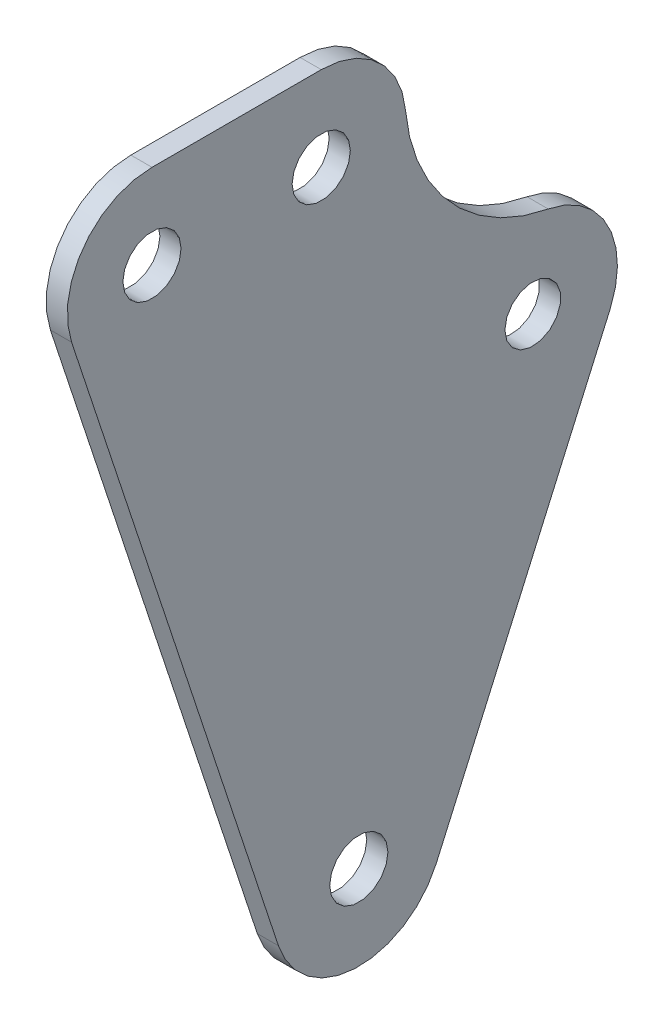
# Autodesk Inventor part: bottom_joint_gusset
Saved by Autodesk Inventor 2025 (Build 290162000, 162)
## iProperties
Created: 2024-10-13
Part Number: bottom_joint_gusset
Material: Generic
Document SubType Name: Modeling
Designer: Averey Ku
Density: 1 g/cm^3
Appearance: Default
Author: Averey Ku
Autodesk Inventor part; units mm, degrees
ref_plane "YZ Plane" through (0, 0, 0) normal (1, 0, 0) x (0, 1, 0)
ref_plane "XZ Plane" through (0, 0, 0) normal (0, 1, 0) x (-1, 0, 0)
ref_plane "XY Plane" through (0, 0, 0) normal (0, 0, 1) x (1, 0, 0)
sketch "maiin" plane through (0, 0, 0) normal (0, 0, 1) x (1, 0, 0)
  circle A0 centre (-0.0182, -20.0228) radius 2.1844
  circle A1 centre (12.6818, -20.0228) radius 2.1844
  circle A2 centre (-2.8225, 26.9672) radius 2.1844 construction
  arc A3 (-6.3396, -20.5787) -> (-0.0224, -26.3686) centre (-0.0182, -20.0228) ccw
  arc A4 (12.6776, -26.377) -> (18.7159, -18.0313) centre (12.6818, -20.0228) ccw
  arc A5 (3.2076, 28.9574) -> (-8.6291, 29.5373) centre (-2.8225, 26.9672) ccw
  arc A6 (-21.694, 0.0193) -> (-17.0461, -8.7942) centre (-15.8874, -2.5508) ccw
  circle A7 centre (-15.8874, -2.5508) radius 2.0955
  line L0 (18.7159, -18.0313) -> (3.2076, 28.9574)
  line L1 (12.6776, -26.377) -> (-0.0224, -26.3686)
  line L2 (-8.6291, 29.5373) -> (-21.694, 0.0193)
  circle A8 centre (-2.8225, 26.9672) radius 2.1844
  arc A9 (-6.3396, -20.5787) -> (-17.0461, -8.7942) centre (-19.447, -21.7313) ccw
  point P0 (3.1417, -3.9392)
  dimension "d0" = 12.7
  dimension "d1" = 12.7
  dimension "d2" = 4.191
  dimension "d3" = 4.3688
  dimension "d7" = 46.99
  measures "d0" diameter of A5
  measures "d1" diameter of A6
  measures "d2" diameter of A7
  measures "d3" diameter of A8
  measures "d7" vertical distance of A2.centre A0.centre
sketch "Sketch1" plane through (0, 0, 0) normal (1, 0, 0) x (0, 1, 0)
  circle A0 centre (0.0042, -12.7) radius 2.1844
  circle A1 centre (0, 0) radius 2.1844
  circle A2 centre (-46.9848, -15.5199) radius 2.1844 construction
  arc A3 (0.5622, -19.0212) -> (6.35, -12.7021) centre (0.0042, -12.7) ccw
  arc A4 (6.3542, -0.0021) -> (-1.9935, 6.0334) centre (0, 0) ccw
  arc A5 (-48.977, -9.4905) -> (-49.553, -21.3275) centre (-46.9848, -15.5199) ccw
  arc A6 (-20.0306, -34.3825) -> (-11.2187, -29.7316) centre (-17.4625, -28.575) ccw
  circle A7 centre (-17.4625, -28.575) radius 2.0955
  line L0 (-1.9935, 6.0334) -> (-48.977, -9.4905)
  line L1 (6.3542, -0.0021) -> (6.35, -12.7021)
  line L2 (-49.553, -21.3275) -> (-20.0306, -34.3825)
  circle A8 centre (-46.9848, -15.5199) radius 2.1844
  arc A9 (0.5622, -19.0212) -> (-11.2187, -29.7316) centre (1.7192, -32.1283) ccw
  point P0 (0, 0)
  constraints: 1 other
extrude "Extrusion1" add sketch "Sketch1" along normal blind 1.5875
body "Solid1"
